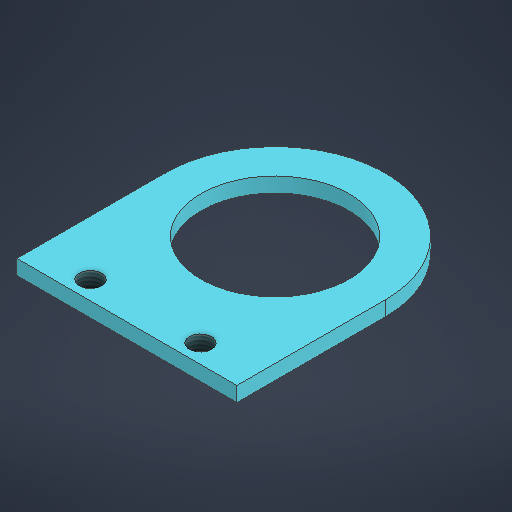
# Autodesk Inventor part: Holder Cover
Saved by Autodesk Inventor 2026.1 (Build 301233000, 233)
## iProperties
Created: 2026-07-20
Part Number: Holder Cover
Material: Generic
Document SubType Name: Modeling
Designer: ankit
Density: 1 g/cm^3
Appearance: Default
Author: ankit
Autodesk Inventor part; units mm, degrees
ref_plane "YZ Plane" through (0, 0, 0) normal (1, 0, 0) x (0, 1, 0)
ref_plane "XZ Plane" through (0, 0, 0) normal (0, 1, 0) x (-1, 0, 0)
ref_plane "XY Plane" through (0, 0, 0) normal (0, 0, 1) x (1, 0, 0)
sketch "Sketch1" plane through (0, 0, 0) normal (0, 1, 0) x (-1, 0, 0)
  arc A0 (-14.8294, -2.4305) -> (14.8706, -2.4305) centre (0.0206, -2.4305) ccw
  line L0 (14.8706, 17.5695) -> (-14.8294, 17.5695)
  line L1 (14.8706, -2.4305) -> (14.8706, 17.5695)
  line L2 (14.8706, 17.5695) -> (-14.8294, 17.5695)
  line L3 (-14.8294, 17.5695) -> (-14.8294, -2.4305)
  circle A1 centre (0.0206, -2.4305) radius 10
  line L4 (0.0206, 17.5695) -> (0.0206, 7.5695)
  line L5 (0.0206, 17.5695) -> (0.0206, 15.0695)
  line L6 (-14.8294, 15.0695) -> (0.0206, 15.0695)
  line L7 (1.5206, 17.5695) -> (1.5206, 12.5695)
  line L8 (0.0206, 15.0695) -> (14.8706, 15.0695)
  circle A2 centre (-7.4044, 15.0695) radius 1.5
  circle A3 centre (7.4456, 15.0695) radius 1.5
  point P0 (0, 0)
  dimension "d0" = 20
  dimension "d1" = 3
  dimension "d2" = 3
  constraints: 18 end point, 4 point on line, 3 centre point, 3 midpoint, 2 coincident, 2 point on circle, 1 parallel, 1 perpendicular, 1 vertical alignment, 2 other
  measures "d1" diameter of A2
  measures "d2" diameter of A3
extrude "Extrusion1" add sketch "Sketch1" along normal blind 2 contours L3 L6 A2 L8 A3 L1 A0 | L3 L0 L4 L6 A2 | L8 A3 L7 L0 L1 | L0 L7 L8 L4
thread "Thread1" size "M3x0.5" class "6H" standard "ANSI Metric M Profile" full length
thread "Thread2" size "M3x0.5" class "6H" standard "ANSI Metric M Profile" full length
body "Solid1"
